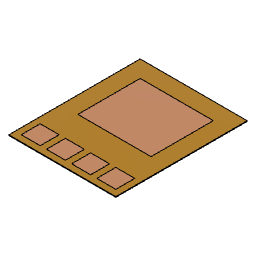
Bx-350-3EB (Autodesk Fusion 360 design; units mm, degrees)
Autodesk Fusion 360 part; units mm, degrees
sketch "Sketch1" plane through (0, 0, 0) normal (0, 0, 1) x (1, 0, 0) in component "Bx-350-3EB"
  line L0 (3.95, -4.85) -> (-3.95, -4.85)
  line L1 (-3.95, -4.85) -> (-3.95, 4.85)
  line L2 (-3.95, 4.85) -> (3.95, 4.85)
  line L3 (3.95, 4.85) -> (3.95, -4.85)
  line L4 (3.95, -4.85) -> (-3.95, 4.85) construction
  line L5 (-3.95, -4.85) -> (3.95, 4.85) construction
  line L6 (0, 0) -> (0, 1.3)
  line L7 (2.7, -1) -> (-2.7, -1)
  line L8 (-2.7, -1) -> (-2.7, 3.6)
  line L9 (-2.7, 3.6) -> (2.7, 3.6)
  line L10 (2.7, 3.6) -> (2.7, -1)
  line L11 (2.7, -1) -> (-2.7, 3.6) construction
  line L12 (-2.7, -1) -> (2.7, 3.6) construction
  line L13 (-3.49, -4.39) -> (-2.09, -4.39)
  line L14 (-2.09, -4.39) -> (-2.09, -2.99)
  line L15 (-2.09, -2.99) -> (-3.49, -2.99)
  line L16 (-3.49, -2.99) -> (-3.49, -4.39)
  line L17 (-1.63, -2.99) -> (-0.23, -2.99)
  line L18 (-0.23, -2.99) -> (-0.23, -4.39)
  line L19 (-0.23, -4.39) -> (-1.63, -4.39)
  line L20 (-1.63, -4.39) -> (-1.63, -2.99)
  line L21 (3.49, -2.99) -> (3.49, -4.39)
  line L22 (3.49, -4.39) -> (2.09, -4.39)
  line L23 (2.09, -4.39) -> (2.09, -2.99)
  line L24 (2.09, -2.99) -> (3.49, -2.99)
  line L25 (0.23, -2.99) -> (0.23, -4.39)
  line L26 (0.23, -4.39) -> (1.63, -4.39)
  line L27 (1.63, -2.99) -> (0.23, -2.99)
  line L28 (1.63, -4.39) -> (1.63, -2.99)
  point P0 (0, 1.3)
  dimension "d1" = 7.9
  dimension "d2" = 9.7
  dimension "d5" = 5.4
  dimension "d6" = 4.6
  dimension "d7" = 1.25
  dimension "d9" = 1.4
  dimension "d10" = 1.4
  dimension "d11" = 1.4
  dimension "d12" = 1.4
  dimension "d13" = 1.4
  dimension "d14" = 1.4
  dimension "d15" = 1.4
  dimension "d16" = 1.4
  dimension "d17" = 0.46
  dimension "d18" = 0.46
  dimension "d19" = 0.46
  dimension "d20" = 0.46
  dimension "d21" = 0.46
  dimension "d26" = 1.25
  dimension "d27" = 0.46
  constraint horizontal L0
  constraint perpendicular L0 L1
  constraint parallel L0 L2
  constraint parallel L1 L3
  constraint coincident L4 L6.start
  constraint coincident L5 L6.start
  constraint coincident L6.start origin
  constraint vertical L6
  constraint horizontal L7
  constraint perpendicular L7 L8
  constraint parallel L7 L9
  constraint parallel L8 L10
  constraint coincident L11 P0
  constraint coincident L12 P0
  constraint coincident P0 L6.end
  constraint horizontal L13
  constraint vertical L14
  constraint horizontal L15
  constraint vertical L16
  constraint horizontal L17
  constraint vertical L18
  constraint horizontal L19
  constraint vertical L20
  constraint horizontal L26
  constraint vertical L28
  constraint horizontal L27
  constraint vertical L25
  constraint horizontal L24
  constraint vertical L21
  constraint horizontal L22
  constraint vertical L23
  constraint coincident L13 L19.end
  constraint coincident L19 L25.end
  constraint coincident L22.end L26
  measures "d1" distance of L1.end L2.end
  measures "d2" distance of L0.end L1.end
  measures "d5" distance of L8.end L9.end
  measures "d6" distance of L7.end L8.end
  measures "d7" distance of L3 L10
  measures "d9" distance of L13.start L13.end
  measures "d10" distance of L13.start L15.end
  measures "d11" distance of L17.start L17.end
  measures "d12" distance of L17.start L19.end
  measures "d13" distance of L26.end L25.end
  measures "d14" distance of L25.start L25.end
  measures "d15" distance of L21.start L23.end
  measures "d16" distance of L22.end L23.end
  measures "d17" distance of L1 L16
  measures "d18" distance of L14 L20
  measures "d19" distance of L18 L25
  measures "d20" distance of L23 L28
  measures "d21" distance of L0 L22
  measures "d26" distance of L2 L9
  measures "d27" distance of L3 L21
extrude "Extrude1" add sketch "Sketch1" against normal blind 0.05 contours L0 L1 L2 L3 | L7 L8 L9 L10 | L13 L14 L15 L16 | L17 L18 L19 L20 | L21 L22 L23 L24 | L25 L26 L27 L28 makes body 1 in component "Bx-350-3EB"
extrude "Extrude2" add sketch "Sketch1" along normal blind 0.005 separate body contours L7 L8 L9 L10 | L13 L14 L15 L16 | L17 L18 L19 L20 | L21 L22 L23 L24 | L25 L26 L27 L28 makes body 2 at (-0.9, 2.0667, 0) makes body 3 at (-3.0233, -3.4567, 0) makes body 4 at (0.6967, -3.9233, 0) makes body 5 at (-1.1633, -3.4567, 0) makes body 6 at (3.0233, -3.4567, 0) in component "Bx-350-3EB"
component "Bx-350-3EB" placed x (1, 0, 0) y (0, 1, 0) z (0, 0, 1) at (0, 0, 0)
equation "d5 = ( 2.7 * 2 ) * 1 mm"
equation "d6 = ( 2.3 * 2 ) * 1 mm"
equation "d17 = ( ( 7.9 - ( 1.4 * 4 ) ) / 5 ) * 1 mm"
equation "d18 = ( ( 7.9 - ( 1.4 * 4 ) ) / 5 ) * 1 mm"
equation "d19 = ( ( 7.9 - ( 1.4 * 4 ) ) / 5 ) * 1 mm"
equation "d20 = ( ( 7.9 - ( 1.4 * 4 ) ) / 5 ) * 1 mm"
equation "d21 = ( ( 7.9 - ( 1.4 * 4 ) ) / 5 ) * 1 mm"
